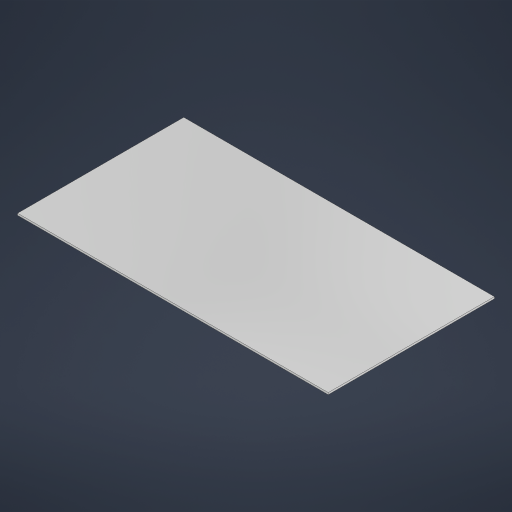
# Autodesk Inventor part: Base Plate
Saved by Autodesk Inventor 2024 (Build 280153000, 153)
## iProperties
Created: 2024-10-26
Part Number: Base Plate
Material: Generic
Document SubType Name: Modeling
Designer: jerem
Density: 1 g/cm^3
Appearance: Default
Author: jerem
Autodesk Inventor part; units mm, degrees
ref_plane "YZ Plane" through (0, 0, 0) normal (1, 0, 0) x (0, 1, 0)
ref_plane "XZ Plane" through (0, 0, 0) normal (0, 1, 0) x (-1, 0, 0)
ref_plane "XY Plane" through (0, 0, 0) normal (0, 0, 1) x (1, 0, 0)
sketch "Sketch1" plane through (0, 0, 0) normal (0, 1, 0) x (-1, 0, 0)
  line L0 (-546.1, -292.1) -> (546.1, -292.1)
  line L1 (546.1, -292.1) -> (546.1, 292.1)
  line L2 (546.1, 292.1) -> (-546.1, 292.1)
  line L3 (-546.1, 292.1) -> (-546.1, -292.1)
  line L4 (-546.1, -292.1) -> (546.1, 292.1) construction
  line L5 (546.1, -292.1) -> (-546.1, 292.1) construction
  point P0 (0, 0)
  dimension "d0" = 1092.2
  dimension "d1" = 584.2
  constraints: 12 end point, 2 midpoint, 2 parallel, 1 horizontal, 1 perpendicular
  measures "d0" distance of L2.end L1.end
  measures "d1" distance of L1.end L0.end
extrude "Extrusion1" add sketch "Sketch1" along normal blind 6.5
body "Solid1"
